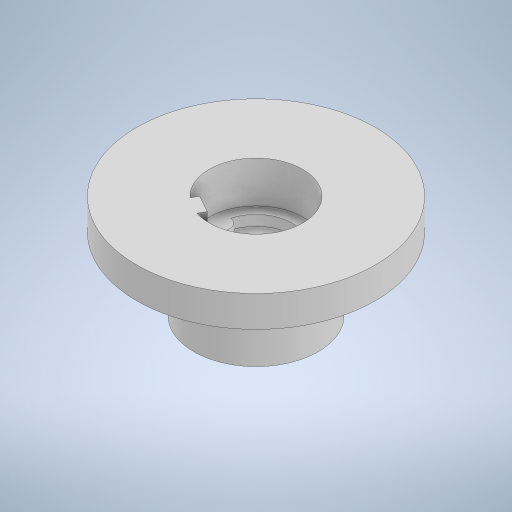
# Autodesk Inventor part: крышка для втулки
Saved by Autodesk Inventor 2023 (Build 270158000, 158)
## iProperties
Created: 2023-04-09
Part Number: крышка для втулки
Material: Типовые
Document SubType Name: Modeling
Designer: deryu
Density: 1 g/cm^3
Appearance: По умолчанию
Author: deryu
Autodesk Inventor part; units mm, degrees
ref_plane "YZ Plane" through (0, 0, 0) normal (1, 0, 0) x (0, 1, 0)
ref_plane "XZ Plane" through (0, 0, 0) normal (0, 1, 0) x (-1, 0, 0)
ref_plane "XY Plane" through (0, 0, 0) normal (0, 0, 1) x (1, 0, 0)
sketch "Эскиз1" plane through (0, 0, 0) normal (0, 1, 0) x (-1, 0, 0)
  circle A0 centre (0, 0) radius 3.5
  circle A1 centre (3.5, 0) radius 0.95
  circle A2 centre (-1.75, 3.0311) radius 0.95
  circle A3 centre (-1.75, -3.0311) radius 0.95
  circle A4 centre (0, 0) radius 4.5
  circle A5 centre (0, 0) radius 1.5
  point P0 (-2.5006, -2.4488)
  point P1 (-2.5006, 2.4488)
  point P2 (-0.8704, 3.39)
  point P3 (3.3711, 0.9412)
  point P4 (3.3711, -0.9412)
  point P5 (-0.8704, -3.39)
  dimension "d0" = 7
  dimension "d1" = 1.9
  dimension "d4" = 360
  dimension "d6" = 9
  dimension "d7" = 3
  constraints: 5 centre point, 3 coincident, 10 other
  measures "d1" diameter of A1
  measures "d6" diameter of A4
  measures "d7" diameter of A5
extrude "Выдавливание1" add sketch "Эскиз1" along normal blind 1 contours A0 A1 | A0 A1 | A2 A0 | A0 A2 | A3 A0 | A0 A3 | A4
sketch "Эскиз2" plane through (0, 0, 0) normal (0, -1, 0) x (1, 0, 0)
  circle A0 centre (0, 0) radius 1.5
  circle A1 centre (0, 0) radius 6
  dimension "d10" = 3
  dimension "d11" = 12
  constraints: 2 centre point, 2 coincident
  measures "d10" diameter of A0
  measures "d11" diameter of A1
extrude "Выдавливание2" add sketch "Эскиз2" along normal blind 5
sketch "Эскиз3" plane through (0, 0, 0) normal (0, 1, 0) x (1, 0, 0)
  circle A0 centre (0, 0) radius 4.5
  circle A1 centre (0, 0) radius 6
  circle A2 centre (0, 0) radius 4.5
  dimension "d14" = 12
  constraints: 3 centre point, 3 coincident
  measures "d14" diameter of A1
extrude "Выдавливание3" add sketch "Эскиз3" along normal blind 5
sketch "Эскиз4" plane through (0, 5, 0) normal (0, 1, 0) x (1, 0, 0)
  arc A0 (0.8704, 3.39) -> (2.5006, 2.4488) centre (1.75, 3.0311) ccw projected
  line L0 (0, 0) -> (1.75, 3.0311)
  line L1 (0, 0) -> (-5.8023, -10.0499)
  line L2 (-3.2807, -7.6668) -> (-1.0566, -3.645)
  line L3 (-1.0566, -3.645) -> (-2.7193, -2.7255)
  line L4 (-2.7193, -2.7255) -> (-4.9434, -6.7473)
  line L5 (-4.9434, -6.7473) -> (-3.2807, -7.6668)
  circle A1 centre (0, 0) radius 6 projected
  line L6 (-3.2807, -7.6668) -> (-2.7193, -2.7255) construction
  line L7 (-1.0566, -3.645) -> (-4.9434, -6.7473) construction
  point P0 (-3, -5.1962)
  point P1 (-2.1406, -5.6052)
  point P2 (-3.7861, -4.6546)
  dimension "d17" = 1.9
  constraints: 16 end point, 2 midpoint, 2 parallel, 1 perpendicular, 1 point on line, 2 other
  measures "d17" distance of L3.end L2.end
extrude "Выдавливание4" add sketch "Эскиз4" against normal blind 5 contours L3 L2 A1 L1 | L1 A1 L4 L3
sketch "Эскиз5" plane through (0, 5, 0) normal (0, 1, 0) x (1, 0, 0)
  circle A0 centre (0, 0) radius 11.5
  circle A1 centre (0, 0) radius 6
  dimension "d20" = 23
  constraints: 2 centre point, 2 coincident
  measures "d20" diameter of A0
extrude "Выдавливание5" add sketch "Эскиз5" against normal blind 3
